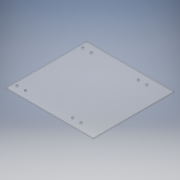
# Autodesk Inventor part: PaddleCollectionFloor
Saved by Autodesk Inventor 2019 (Build 230136000, 136)
## iProperties
Created: 2018-10-18
Part Number: PaddleCollectionFloor
Material: Polycarbonate, Clear
Document SubType Name: Modeling
Designer: User
Density: 1.2 g/cm^3
Appearance: Polycarbonate - Clear
Mass: 55.9848 g
Surface Area: 514.999 cm^2
Volume: 46.654 cm^3
Author: User
Autodesk Inventor part; units mm, degrees
ref_plane "YZ Plane" through (0, 0, 0) normal (1, 0, 0) x (0, 1, 0)
ref_plane "XZ Plane" through (0, 0, 0) normal (0, 1, 0) x (-1, 0, 0)
ref_plane "XY Plane" through (0, 0, 0) normal (0, 0, 1) x (1, 0, 0)
sketch "Sketch1" plane through (0, 0, 0) normal (0, 1, 0) x (-1, 0, 0)
  line L0 (0, 0) -> (165.1, 0)
  line L1 (165.1, 0) -> (165.1, -152.4)
  line L2 (165.1, -152.4) -> (0, -152.4)
  line L3 (0, -152.4) -> (0, 0)
  dimension "d0" = 165.1
  dimension "d1" = 152.4
  constraints: 8 end point, 2 parallel, 1 horizontal, 1 perpendicular
  measures "d0" distance of L1.end L2.end
  measures "d1" distance of L0.end L1.end
extrude "Extrusion1" add sketch "Sketch1" along normal blind 1.8542
sketch "Sketch2" plane through (0, 1.8542, 0) normal (0, 1, 0) x (1, 0, 0)
  line L0 (-165.1, 0) -> (0, 0) projected
  line L1 (0, 0) -> (0, 152.4) projected
  line L2 (0, 152.4) -> (-165.1, 152.4) projected
  line L3 (-165.1, 152.4) -> (-165.1, 0) projected
  point P0 (-158.242, 14.1478)
  point P1 (-142.242, 14.1478)
  point P2 (-53.2638, 14.1478)
  point P3 (-37.2638, 14.1478)
  point P4 (-37.2638, 138.2522)
  point P5 (-53.2638, 138.2522)
  point P6 (-142.242, 138.2522)
  point P7 (-158.242, 138.2522)
  dimension "d4" = 165.1
  dimension "d5" = 16
  dimension "d6" = 16
  dimension "d7" = 16
  dimension "d8" = 16
  dimension "d9" = 14.1478
  dimension "d10" = 14.1478
  dimension "d11" = 14.1478
  dimension "d12" = 14.1478
  dimension "d13" = 14.1478
  dimension "d14" = 14.1478
  dimension "d15" = 14.1478
  dimension "d16" = 14.1478
  dimension "d17" = 53.2638
  dimension "d18" = 53.2638
  dimension "d19" = 158.242
  dimension "d20" = 158.242
  measures "d4" distance of L1.end L2.end
  measures "d5" distance of point (-142.242, 138.252) point (-158.242, 138.252)
  measures "d6" distance of point (-37.264, 138.252) point (-53.264, 138.252)
  measures "d7" distance of point (-158.242, 14.148) point (-142.242, 14.148)
  measures "d8" distance of point (-37.264, 14.148) point (-53.264, 14.148)
  measures "d9" distance from line of L2 point (-158.242, 138.252)
  measures "d10" distance from line of L2 point (-142.242, 138.252)
  measures "d11" distance from line of L2 point (-53.264, 138.252)
  measures "d12" distance from line of L2 point (-37.264, 138.252)
  measures "d13" distance from line of L0 point (-158.242, 14.148)
  measures "d14" distance from line of L0 point (-142.242, 14.148)
  measures "d15" distance from line of L0 point (-53.264, 14.148)
  measures "d16" distance from line of L0 point (-37.264, 14.148)
  measures "d17" distance from line of L1 point (-53.264, 138.252)
  measures "d18" distance from line of L1 point (-53.264, 14.148)
  measures "d19" distance from line of L1 point (-158.242, 138.252)
  measures "d20" distance from line of L1 point (-158.242, 14.148)
hole "Hole1" at (-158.242, 1.8542, -14.1478) at (-142.242, 1.8542, -14.1478) at (-53.2638, 1.8542, -14.1478) at (-37.2638, 1.8542, -14.1478) at (-37.2638, 1.8542, -138.2522) at (-53.2638, 1.8542, -138.2522) at (-142.242, 1.8542, -138.2522) at (-158.242, 1.8542, -138.2522) direction (0, -1, 0) diameter 3.81 depth 10.9728 tip angle 118
equation "\"d6\" = d5"
equation "\"d7\" = d5"
equation "\"d8\" = d5"
equation "\"d10\" = d9"
equation "\"d11\" = d9"
equation "\"d12\" = d9"
equation "\"d13\" = d9"
equation "\"d14\" = d9"
equation "\"d15\" = d9"
equation "\"d16\" = d9"
equation "\"d18\" = d17"
equation "\"d20\" = d19"
body "Solid1"
